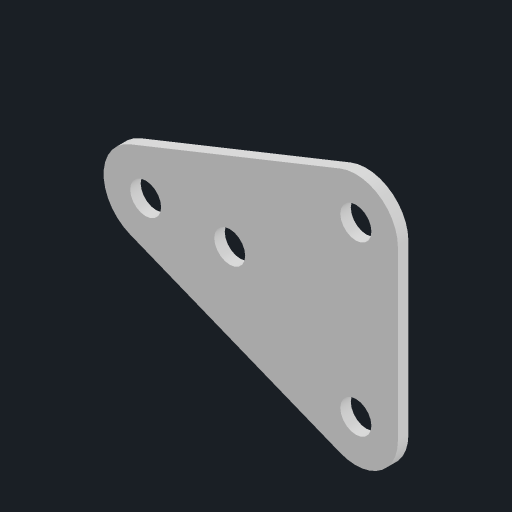
# Autodesk Inventor part: imuMount
Saved by Autodesk Inventor 2024.2 (Build 282272000, 272)
## iProperties
Created: 2024-01-29
Part Number: imuMount
Material: Generic
Document SubType Name: Sheet Metal
Designer: reima
Density: 1 g/cm^3
Sheet Metal Rule: Default
Appearance: Default
Author: reima
Autodesk Inventor part; units mm, degrees
ref_plane "YZ Plane" through (0, 0, 0) normal (1, 0, 0) x (0, 1, 0)
ref_plane "XZ Plane" through (0, 0, 0) normal (0, 1, 0) x (-1, 0, 0)
ref_plane "XY Plane" through (0, 0, 0) normal (0, 0, 1) x (1, 0, 0)
sketch "Sketch1" plane through (0, 0, 0) normal (0, 0, 1) x (1, 0, 0)
  circle A0 centre (0.7751, 12.7) radius 2.1844 construction
  circle A1 centre (0.7751, -12.7) radius 2.1844 construction
  circle A2 centre (0.7751, 12.7) radius 2.3495
  circle A3 centre (0.7751, -12.7) radius 2.3495
  circle A4 centre (-18.2749, 0) radius 2.3368
  circle A5 centre (-30.9749, 0) radius 2.3368
  circle A6 centre (-30.9749, 0) radius 6.35
  circle A7 centre (0.7751, -12.7) radius 6.35
  circle A8 centre (0.7751, 12.7) radius 6.35
  line L0 (7.1251, 12.7) -> (7.1251, -12.7)
  line L1 (-1.5832, -18.5958) -> (-33.3332, -5.8958)
  line L2 (-1.5832, 18.5958) -> (-33.3332, 5.8958)
  point P0 (0, 0)
  dimension "d0" = 4.699
  dimension "d1" = 4.699
  dimension "d2" = 4.6736
  dimension "d3" = 4.6736
  dimension "d4" = 12.7
  dimension "d5" = 19.05
  dimension "d6" = 12.7
  dimension "d7" = 12.7
  dimension "d8" = 12.7
  constraints: 7 centre point, 6 end point, 6 point on circle, 6 tangent, 5 coincident
  measures "d0" diameter of A2
  measures "d1" diameter of A3
  measures "d2" diameter of A4
  measures "d3" diameter of A5
  measures "d4" distance of A5.centre A4.centre
  measures "d5" horizontal distance of A1.centre A4.centre
  measures "d6" diameter of A6
  measures "d7" diameter of A7
  measures "d8" diameter of A8
extrude "Plate1" add sketch "Sketch1" along normal blind 1.5875 contours A6 | A6 L2 A8 L0 A7 L1
sheet face with bend "Face2" sketch "Sketch1" thickness 1.5875 toward (0, 0, 1) bend radius 1.5875 contours A8 | A7
bend "Bend1"
equation "\"d9\" = Thickness"
equation "\"d10\" = BendRadius"
equation "\"d11\" = BendReliefWidth"
equation "\"d13\" = MinimumRemnant"
equation "\"d12\" = BendReliefDepth"
equation "\"d14\" = TransitionRadius"
equation "\"BendRadius\" = Thickness"
equation "\"BendReliefWidth\" = Thickness"
equation "\"BendReliefDepth\" = 0.5 * Thickness"
equation "\"CornerReliefSize\" = 4 * Thickness"
equation "\"MinimumRemnant\" = 2 * Thickness"
equation "\"TransitionRadius\" = BendRadius"
equation "\"JacobiRadiusSize\" = BendRadius"
equation "\"GapSize\" = Thickness"
equation "\"Thickness\" = 1.5875"
body "Solid1"
